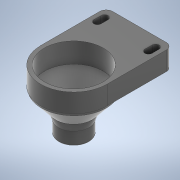
# Autodesk Inventor part: Chute
Saved by Autodesk Inventor 2020.2 (Build 242310000, 310)
## iProperties
Created: 2020-10-16
Part Number: Chute
Material: Generic
Document SubType Name: Modeling
Designer: JK
Density: 1 g/cm^3
Appearance: Smooth - Black
Author: JK
Autodesk Inventor part; units mm, degrees
ref_plane "YZ Plane" through (0, 0, 0) normal (1, 0, 0) x (0, 1, 0)
ref_plane "XZ Plane" through (0, 0, 0) normal (0, 1, 0) x (-1, 0, 0)
sketch "Sketch1" plane through (0, 0, 0) normal (0, 1, 0) x (-1, 0, 0)
  circle A0 centre (0, 0) radius 10.3
  circle A1 centre (0, 0) radius 13.3
  dimension "d0" = 20.6
  dimension "d1" = 3
  constraints: 2 centre point, 2 coincident
  measures "d0" diameter of A0
  measures "d1" radial gap between concentric circles of A1 A0
extrude "Extrusion1" add sketch "Sketch1" along normal blind 25
sketch "Sketch2" plane through (0, 0, 0) normal (0, 0, 1) x (1, 0, 0)
  circle A0 centre (0, 4) radius 16
  line L0 (13.3, 25) -> (-13.3, 25) projected
  line L1 (0, 25) -> (0, 20)
  point P0 (0, 0)
  dimension "d4" = 32
  dimension "d5" = 5
  constraints: 2 end point, 2 vertical alignment, 1 midpoint, 1 perpendicular, 2 other
  measures "d5" distance of L1.start L1.end
extrude "Extrusion2" cut sketch "Sketch2" against normal through all both and the other way through all
sketch "Sketch4" plane through (0, 0, 0) normal (1, 0, 0) x (0, 1, 0)
  line L0 (20, 13.3) -> (25, 13.3) projected
  line L1 (25, 13.3) -> (40, 25.6)
  line L2 (40, 25.6) -> (55, 25.6)
  line L3 (55, 25.6) -> (55, 22.6)
  line L4 (55, 22.6) -> (40, 22.6)
  line L5 (25, 10.3) -> (25, -10.3) projected
  line L6 (40, 22.6) -> (25, 10.3)
  line L7 (0, 0) -> (85.2959, 0)
  line L8 (25, 13.3) -> (25, 10.3)
  line L9 (25, -13.3) -> (25, 13.3) projected
  point P0 (25, 0)
  dimension "d8" = 22.6
  dimension "d9" = 3
  dimension "d11" = 15
  dimension "d12" = 30
  constraints: 14 end point, 2 parallel, 2 perpendicular, 1 collinear, 1 horizontal, 1 midpoint, 1 point on line, 1 vertical alignment
  measures "d8" vertical distance of L3.end point (25, 0)
  measures "d9" distance between parallel lines of L4 L2
  measures "d11" horizontal distance of L4.end point (25, 0)
  measures "d12" horizontal distance of point (25, 0) L3.end
revolve "Revolution1" add sketch "Sketch4" angle 360 about axis through (0, 0, 0) along (0, 1, 0)
chamfer "Chamfer1" distance 1 angle 45 5 edges at (0, 40, -25.6) (0, 55, -22.6) (10.3, 16.2438, -0.0012) (9.4045, 25, -9.4045) (-9.4045, 25, 9.4045)
sketch "Sketch5" plane through (0, 0, 0) normal (0, 1, 0) x (-1, 0, 0)
  circle A0 centre (0, 0) radius 13.9341 projected
  circle A1 centre (0, 0) radius 35.7982
  point P0 (0, 0)
  constraints: 1 centre point, 1 coincident
extrude "Extrusion3" cut sketch "Sketch5" along normal blind 24 contours A0 | A1
sketch "Sketch6" plane through (0, 24, 0) normal (0, -1, 0) x (1, 0, 0)
  circle A0 centre (0, 0) radius 10.3
  circle A1 centre (0, 0) radius 13.3
  constraints: 2 centre point, 2 coincident
extrude "Extrusion4" add sketch "Sketch6" along normal blind 10
sketch "Sketch7" plane through (0, 14, 0) normal (0, -1, 0) x (1, 0, 0)
  circle A0 centre (0, 0) radius 6.75
  circle A1 centre (0, 0) radius 13.3 projected
  circle A2 centre (0, 0) radius 10.3 projected
  dimension "d21" = 13.5
  constraints: 1 centre point, 1 coincident
  measures "d21" diameter of A0
extrude "Extrusion5" add sketch "Sketch7" against normal blind 11 contours A1 | A2
fillet "Fillet1" radius 2 1 edges at (-6.75, 14, 0)
sketch "Sketch8" plane through (0, 55, 0) normal (0, 1, 0) x (1, 0, 0)
  circle A0 centre (0, 0) radius 22.8
  dimension "d28" = 45.6
  constraints: 1 centre point, 1 coincident
  measures "d28" diameter of A0
extrude "Extrusion6" cut sketch "Sketch8" against normal blind 15
sketch "Sketch10" plane through (0, 55, 0) normal (0, 1, 0) x (1, 0, 0)
  line L0 (-37.6, 25.6) -> (37.6, 25.6)
  line L1 (37.6, 25.6) -> (37.6, 0)
  line L2 (37.6, 0) -> (-37.6, 0)
  line L3 (-37.6, 0) -> (-37.6, 25.6)
  circle A0 centre (0, 0) radius 25.6 projected
  circle A1 centre (0, 0) radius 25.6 projected
  point P0 (-25.6, 0)
  point P1 (25.6, 0)
  point P2 (0, 25.6)
  point P3 (25.6, 0)
  dimension "d34" = 12
  dimension "d35" = 12
  constraints: 8 end point, 2 parallel, 2 point on line, 1 horizontal, 1 perpendicular, 1 point on circle, 1 tangent, 2 other
  measures "d34" distance from line of L3 A1.start
  measures "d35" distance from line of L1 A1.end
extrude "Extrusion8" add sketch "Sketch10" against normal blind 14 contours L0 A0 L2 L3 | L0 L1 L2 A0
sketch "Sketch11" plane through (-37.6, 55, -25.6) normal (0, 1, 0) x (1, 0, 0)
  line L0 (0, -25.6) -> (12, -25.6) projected
  line L1 (75.2, 0) -> (0, 0) projected
  line L2 (12, -25.6) -> (0, 0)
  line L3 (0, 0) -> (0, -25.6)
  arc A0 (12, -25.6) -> (63.2, -25.6) centre (37.6, -25.6) ccw projected
  line L4 (12, -25.6) -> (0, -25.6)
  arc A1 (63.2, -25.6) -> (37.6, 0) centre (37.6, -25.6) ccw projected
  line L5 (63.2, -25.6) -> (75.2, 0)
  line L6 (63.2, -25.6) -> (75.2, -25.6) projected
  line L7 (63.2, -25.6) -> (75.2, -25.6)
  line L8 (75.2, 0) -> (75.2, -25.6) projected
  line L9 (75.2, -25.6) -> (75.2, 0)
  constraints: 12 end point, 2 collinear, 1 perpendicular, 1 vertical
extrude "Extrusion9" [suppressed]
sketch "Sketch12" plane through (0, 0, 0) normal (0, 0, 1) x (1, 0, 0)
  circle A0 centre (-31.1, 48) radius 4.75
  circle A1 centre (31.1, 48) radius 4.75
  line L0 (-37.6, 55) -> (-37.6, 41) projected
  line L1 (37.6, 55) -> (37.6, 41) projected
  line L2 (37.6, 41) -> (25.6, 41) projected
  point P0 (0, 0)
  dimension "d40" = 9.5
  dimension "d41" = 6.5
  dimension "d42" = 6.5
  dimension "d43" = 7
  constraints: 2 centre point, 1 equal radius, 1 horizontal alignment
  measures "d40" diameter of A0
  measures "d41" distance from line of L0 A0.centre
  measures "d42" distance from line of L1 A1.centre
  measures "d43" distance from line of L2 A1.centre
extrude "Extrusion10" [suppressed]
sketch "Sketch13" plane through (0, 0, -21.6) normal (0, 0, 1) x (1, 0, 0)
  arc A0 (-35.725, 46.9175) -> (-35.725, 49.0825) centre (-31.1, 48) ccw projected
  circle A1 centre (-31.1, 48) radius 2.75
  arc A2 (35.725, 49.0825) -> (35.725, 46.9175) centre (31.1, 48) ccw projected
  circle A3 centre (31.1, 48) radius 2.75
  point P0 (0, 0)
  dimension "d46" = 5.5
  constraints: 2 centre point, 2 coincident, 1 equal radius
  measures "d46" diameter of A1
extrude "Extrusion11" [suppressed]
sketch "Sketch17" plane through (0, 14, 0) normal (0, -1, 0) x (1, 0, 0)
  circle A0 centre (0, 0) radius 10.9341
  circle A1 centre (0, 0) radius 13.9341 projected
  dimension "d53" = 3
  constraints: 1 centre point, 1 coincident
  measures "d53" radial gap between concentric circles of A1 A0
extrude "Extrusion12" cut sketch "Sketch17" against normal through all contours A0
sketch "Sketch18" plane through (0, 14, 0) normal (0, -1, 0) x (1, 0, 0)
  circle A0 centre (0, 0) radius 20.3
  circle A1 centre (0, 0) radius 13.3 projected
  dimension "d56" = 7
  constraints: 1 centre point, 1 coincident
  measures "d56" radial gap between concentric circles of A0 A1
extrude "Extrusion13" add sketch "Sketch18" against normal blind 3
chamfer "Chamfer3" distance 7 angle 45 1 edges at (-13.3, 17, 0)
ref_plane "Work Plane1" through (-37.6, 24, -25.6) normal (0, 1, 0) x (1, 0, 0)
sketch "Sketch20" plane through (-37.6, 24, -25.6) normal (0, 1, 0) x (1, 0, 0)
  circle A0 centre (20.6, -25.6) radius 3
  line L0 (20.6, -29.0641) -> (17.6, -27.3321)
  line L1 (17.6, -27.3321) -> (17.6, -23.8679)
  line L2 (17.6, -23.8679) -> (20.6, -22.1359)
  line L3 (20.6, -22.1359) -> (23.6, -23.8679)
  line L4 (23.6, -23.8679) -> (23.6, -27.3321)
  line L5 (23.6, -27.3321) -> (20.6, -29.0641)
  point P0 (37.6, -25.6)
  dimension "d64" = 6
  dimension "d65" = 17
  constraints: 12 end point, 1 centre point, 1 coincident, 1 horizontal alignment, 1 tangent, 1 vertical alignment, 13 other
  measures "d64" diameter of A0
  measures "d65" distance of A0.centre point (37.6, -25.6)
extrude "Extrusion14" cut sketch "Sketch20" against normal blind 7
sketch "Sketch21" plane through (0, 14, 0) normal (0, -1, 0) x (1, 0, 0)
  circle A0 centre (-17, 0) radius 1.75
  point P0 (0, 0)
  dimension "d68" = 3.5
  dimension "d69" = 17
  constraints: 1 centre point
  measures "d68" diameter of A0
  measures "d69" distance of point (0, 0) A0.centre
extrude "Extrusion15" cut sketch "Sketch21" against normal blind 10
pattern_circular "Circular Pattern1" count 6 over 360 about axis through (0, 47.5, 0) along (0, 1, 0) of "Extrusion15", "Extrusion14"
sketch "Sketch23" plane through (-37.6, 55, -25.6) normal (0, 1, 0) x (1, 0, 0)
  line L0 (75.2, 0) -> (0, 0) projected
  arc A0 (12, -25.6) -> (63.2, -25.6) centre (37.6, -25.6) ccw projected
  circle A1 centre (37.6, -25.6) radius 23.6 projected
  circle A2 centre (37.6, -25.6) radius 22.8 projected
  line L1 (63.2, -25.6) -> (75.2, -25.6) projected
  line L2 (75.2, -25.6) -> (75.2, 0) projected
  line L3 (0, 0) -> (0, -25.6) projected
  line L4 (0, -25.6) -> (12, -25.6) projected
sketch "Sketch24" plane through (-37.6, 55, -25.6) normal (0, 1, 0) x (1, 0, 0)
  circle A0 centre (37.6, -25.6) radius 23.6
  circle A1 centre (37.6, -25.6) radius 23.6 projected
  circle A2 centre (37.6, -25.6) radius 22.8
  circle A3 centre (37.6, -25.6) radius 22.8 projected
  constraints: 2 centre point, 2 coincident, 2 concentric
extrude "Extrusion16" add sketch "Sketch24" against normal blind 2
sketch "Sketch25" plane through (-37.6, 55, -25.6) normal (0, 1, 0) x (1, 0, 0)
  circle A0 centre (37.6, -25.6) radius 22.8 projected
  line L0 (75.2, 0) -> (0, 0) projected
  arc A1 (12, -25.6) -> (63.2, -25.6) centre (37.6, -25.6) ccw projected
  line L1 (63.2, -25.6) -> (75.2, -25.6) projected
  line L2 (75.2, -25.6) -> (75.2, 0) projected
  line L3 (0, 0) -> (0, -25.6) projected
  line L4 (0, -25.6) -> (12, -25.6) projected
extrude "Extrusion17" add sketch "Sketch25" along normal blind 3
sketch "Sketch26" plane through (-37.6, 58, -25.6) normal (0, 1, 0) x (1, 0, 0)
  line L0 (11.9256, -25.6) -> (63.2, -25.6)
  line L1 (63.2, -25.6) -> (63.2, 25)
  line L2 (63.2, 25) -> (11.9256, 25)
  line L3 (11.9256, 25) -> (11.9256, -25.6)
  line L4 (75.2, 0) -> (0, 0) projected
  circle A0 centre (17.9256, 15) radius 2.75
  circle A1 centre (57.2, 15) radius 2.75
  line L5 (37.6, 0) -> (75.2, 0) projected
  line L6 (63.2, 0) -> (11.9256, 0)
  line L7 (0, 0) -> (37.6, 0) projected
  point P0 (37.6, -25.6)
  point P1 (11.9256, 0)
  point P2 (63.2, 0)
  dimension "d79" = 25
  dimension "d80" = 5.5
  dimension "d81" = 6
  dimension "d82" = 6
  dimension "d91" = 15
  constraints: 10 end point, 4 point on line, 2 centre point, 2 parallel, 1 equal radius, 1 horizontal, 1 horizontal alignment, 1 perpendicular
  measures "d79" distance between parallel lines of L2 L4
  measures "d80" diameter of A0
  measures "d81" distance from line of L3 A0.centre
  measures "d82" distance from line of L1 A1.centre
  measures "d91" distance from line of L4 A0.centre
extrude "Extrusion18" add sketch "Sketch26" against normal up to surface (17 mm away) contours L3 L2 L1 L4
sketch "Sketch27" plane through (-37.6, 58, -25.6) normal (0, 1, 0) x (1, 0, 0)
  line L0 (11.9256, 25) -> (11.9256, 0) projected
  line L1 (-19.2052, -40.8404) -> (11.9256, -40.8404)
  line L2 (11.9256, -40.8404) -> (11.9256, 11.2059)
  line L3 (11.9256, 11.2059) -> (-19.2052, 11.2059)
  line L4 (-19.2052, 11.2059) -> (-19.2052, -40.8404)
  line L5 (63.2, 0) -> (63.2, 25) projected
  line L6 (63.2, 17.9527) -> (82.2369, 17.9527)
  line L7 (82.2369, 17.9527) -> (82.2369, -35.178)
  line L8 (82.2369, -35.178) -> (63.2, -35.178)
  line L9 (63.2, -35.178) -> (63.2, 17.9527)
  point P0 (37.6, -25.6)
  constraints: 16 end point, 4 parallel, 2 horizontal, 2 perpendicular, 2 point on line
extrude "Extrusion19" cut sketch "Sketch27" against normal through all
sketch "Sketch28" plane through (-37.6, 58, -25.6) normal (0, 1, 0) x (1, 0, 0)
  line L0 (20.6756, 12.25) -> (15.1756, 12.25)
  line L1 (15.1756, 12.25) -> (15.1756, 17.75)
  line L2 (15.1756, 17.75) -> (20.6756, 17.75)
  line L3 (20.6756, 17.75) -> (20.6756, 12.25)
  circle A0 centre (17.9256, 15) radius 2.75 projected
  line L4 (20.6756, 12.25) -> (15.1756, 17.75) construction
  line L5 (15.1756, 12.25) -> (20.6756, 17.75) construction
  line L6 (59.95, 12.25) -> (54.45, 12.25)
  line L7 (54.45, 12.25) -> (54.45, 17.75)
  line L8 (54.45, 17.75) -> (59.95, 17.75)
  line L9 (59.95, 17.75) -> (59.95, 12.25)
  circle A1 centre (57.2, 15) radius 2.75 projected
  line L10 (59.95, 12.25) -> (54.45, 17.75) construction
  line L11 (54.45, 12.25) -> (59.95, 17.75) construction
  circle A2 centre (17.9256, 12.25) radius 2.75
  circle A3 centre (17.9256, 17.75) radius 2.75
  circle A4 centre (57.2, 12.25) radius 2.75
  circle A5 centre (57.2, 17.75) radius 2.75
  point P0 (37.6, -25.6)
  point P1 (20.6756, 12.25)
  point P2 (20.6756, 17.75)
  dimension "d87" = 5.5
  dimension "d88" = 5.5
  constraints: 24 end point, 8 midpoint, 4 parallel, 2 horizontal, 2 perpendicular, 12 other
  measures "d87" distance of point (17.926, 17.75) point (17.926, 12.25)
  measures "d88" distance of L6.end L7.end
extrude "Extrusion20" cut sketch "Sketch28" against normal through all
sketch "Sketch29" plane through (0, 14, 0) normal (0, -1, 0) x (1, 0, 0)
  circle A0 centre (0, 0) radius 35.383
  constraints: 1 centre point, 1 coincident
extrude "Extrusion21" cut sketch "Sketch29" against normal blind 10
sketch "Sketch31" plane through (0, 0, 0) normal (1, 0, 0) x (0, 1, 0)
  line L0 (24, 13.3) -> (25.7733, 13.9341) projected
  line L1 (24, 13.3) -> (19.5254, 11.7)
  line L2 (10.3519, 0) -> (30.0392, 0)
  line L3 (24, -13.3) -> (24, 13.3) projected
  line L4 (24, 11.7) -> (19.5254, 9.7)
  line L5 (19.5254, 11.7) -> (19.5254, 9.7)
  line L6 (24, 11.7) -> (24, 13.3)
  point P0 (0, 0)
  dimension "d95" = 11.7
  dimension "d96" = 2
  constraints: 10 end point, 3 point on line, 1 collinear, 1 horizontal, 1 horizontal alignment, 1 vertical
  measures "d95" distance from line of L2 L1.end
  measures "d96" distance of L4.end L1.end
revolve "Revolution2" add sketch "Sketch31" angle 360 about axis through (0, 10.3519, 0) along (0, 1, 0)
sketch "Sketch32" plane through (0, 19.5254, 0) normal (0, -1, 0) x (1, 0, 0)
  circle A0 centre (0, 0) radius 9.7 projected
  circle A1 centre (0, 0) radius 11.7 projected
extrude "Extrusion22" add sketch "Sketch32" along normal blind 10
sketch "Sketch33" plane through (-37.6, 58, -25.6) normal (0, 1, 0) x (1, 0, 0)
  circle A0 centre (37.6, -25.6) radius 22.65
  circle A1 centre (37.6, -25.6) radius 22.8
  circle A2 centre (37.6, -25.6) radius 22.8 projected
  dimension "d100" = 45.3
  constraints: 2 centre point, 2 coincident, 1 concentric
  measures "d100" diameter of A0
extrude "Extrusion23" add sketch "Sketch33" against normal blind 18
fillet "Fillet2" radius 5 2 edges at (25.6, 49.5, -50.6) (-25.6744, 49.5, -50.6)
fillet "Fillet3" radius 1 1 edges at (-11.7, 9.5254, 0)
sketch "Sketch34" plane through (-37.6, 58, -25.6) normal (0, 1, 0) x (1, 0, 0)
  line L0 (-0.5139, -99.2858) -> (75.7139, -99.2858)
  line L1 (75.7139, -99.2858) -> (75.7139, 48.0858)
  line L2 (75.7139, 48.0858) -> (-0.5139, 48.0858)
  line L3 (-0.5139, 48.0858) -> (-0.5139, -99.2858)
  line L4 (-0.5139, -99.2858) -> (75.7139, 48.0858) construction
  line L5 (75.7139, -99.2858) -> (-0.5139, 48.0858) construction
  point P0 (37.6, -25.6)
  constraints: 12 end point, 2 midpoint, 2 parallel, 1 horizontal, 1 perpendicular
extrude "Extrusion24" cut sketch "Sketch34" against normal blind 2.5
body "Solid1"
